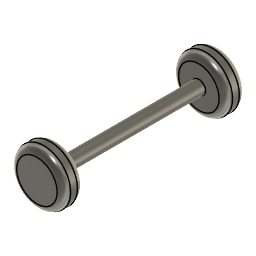
Dozer and Engine Assembly (Autodesk Fusion 360 archive; units mm, degrees)
design "Wheels"
part number: 2026-03-04-16-00-43-502
Autodesk Fusion 360 part; units mm, degrees
note: some values were not read from the file. Set by a fixed rule: which face or edge a step refers to.
sketch "Sketch1" plane through (0, 0, 0) normal (0, 1, 0) x (1, 0, 0)
  circle A0 centre (0, 0) radius 2.54
  dimension "d1" = 5.08
  constraint coincident A0.centre origin
  measures "d1" diameter of A0
extrude "Extrude1" add sketch "Sketch1" along normal mid plane 53.34
sketch "Sketch2" plane through (0, -26.67, 0) normal (0, -1, 0) x (1, 0, 0)
  circle A0 centre (0, 0) radius 2.54
  circle A1 centre (0, 0) radius 10.16
  dimension "d8" = 20.32
  constraint coincident A0.centre A1.centre
  measures "d8" diameter of A1
extrude "Extrude2" add sketch "Sketch2" along normal blind 7.62 contours A0 | A1
sketch "Sketch3" plane through (0, 26.67, 0) normal (0, 1, 0) x (-1, 0, 0)
  circle A0 centre (0, 0) radius 2.54
  circle A1 centre (0, 0) radius 10.16
  dimension "d9" = 20.32
  constraint coincident A0.centre A1.centre
  measures "d9" diameter of A1
extrude "Extrude3" add sketch "Sketch3" along normal blind 7.62 contours A0 | A1
fillet "Fillet1" radius 2.54 3 edges at (-9.4724, -34.29, -3.674) (9.4724, 34.29, -3.674) (-9.4724, -26.67, -3.674) 1 faces at (-10.1474, 29.21, -0.5064)

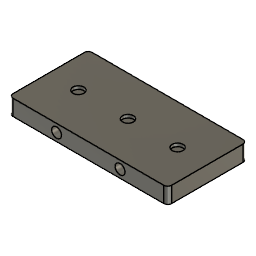
design "Base"
part number: 2026-03-04-09-38-15-257
Autodesk Fusion 360 part; units mm, degrees
sketch "Sketch1" plane through (0, 0, 0) normal (0, 0, 1) x (1, 0, 0)
  line L0 (50.8, -25.4) -> (-50.8, -25.4)
  line L1 (-50.8, -25.4) -> (-50.8, 25.4)
  line L2 (-50.8, 25.4) -> (50.8, 25.4)
  line L3 (50.8, 25.4) -> (50.8, -25.4)
  line L4 (50.8, -25.4) -> (-50.8, 25.4) construction
  line L5 (-50.8, -25.4) -> (50.8, 25.4) construction
  dimension "d2" = 101.6
  dimension "d8" = 50.8
  constraint horizontal L0
  constraint perpendicular L0 L1
  constraint parallel L0 L2
  constraint parallel L1 L3
  constraint coincident L4 origin
  constraint coincident L5 origin
  measures "d2" distance of L1 L3
  measures "d8" distance of L0 L2
extrude "Extrude1" add sketch "Sketch1" against normal blind 10.16
sketch "Sketch2" plane through (0, 0, 0) normal (0, 0, 1) x (-1, 0, 0)
  line L0 (-50.8, -25.4) -> (50.8, -25.4)
  line L1 (50.8, -25.4) -> (50.8, 25.4)
  line L2 (50.8, 25.4) -> (-50.8, 25.4)
  line L3 (-50.8, 25.4) -> (-50.8, -25.4)
  circle A0 centre (31.75, 0) radius 3.5
  circle A1 centre (0, 0) radius 3.5
  circle A2 centre (-31.75, 0) radius 3.5
  line L4 (12.7, -25.4) -> (12.7, 25.4) construction
  dimension "d11" = 7
  dimension "d12" = 19.05
  dimension "d13" = 7
  dimension "d14" = 50.8
  dimension "d15" = 7
  dimension "d16" = 19.05
  dimension "d17" = 25.4
  dimension "d18" = 25.4
  dimension "d19" = 25.4
  dimension "d22" = 38.1
  constraint coincident L0 L4.start
  constraint coincident L2 L4.end
  constraint perpendicular L2 L4
  measures "d11" diameter of A0
  measures "d12" distance of L1 A0.centre
  measures "d13" diameter of A1
  measures "d14" distance of L3 A1.centre
  measures "d15" diameter of A2
  measures "d16" distance of L3 A2.centre
  measures "d17" distance of L2 A0.centre
  measures "d18" distance of L2 A1.centre
  measures "d19" distance of L2 A2.centre
  measures "d22" distance of L1 L4
extrude "Extrude2" cut sketch "Sketch2" against normal blind 2 contours A0 | A1 | A2
sketch "Sketch3" plane through (0, -25.4, 0) normal (0, -1, 0) x (1, 0, 0)
  line L0 (50.8, 0) -> (-50.8, 0)
  line L1 (-50.8, 0) -> (-50.8, -10.16)
  line L2 (-50.8, -10.16) -> (50.8, -10.16)
  line L3 (50.8, -10.16) -> (50.8, 0)
  circle A0 centre (-20.32, -5.08) radius 3.175
  circle A1 centre (20.32, -5.08) radius 3.175
  dimension "d23" = 30.48
  dimension "d24" = 30.48
  dimension "d25" = 6.35
  dimension "d26" = 6.35
  dimension "d27" = 5.08
  dimension "d28" = 5.08
  measures "d23" distance of L1 A0.centre
  measures "d24" distance of L3 A1.centre
  measures "d25" diameter of A0
  measures "d26" diameter of A1
  measures "d27" distance of L0 A0.centre
  measures "d28" distance of L0 A1.centre
extrude "Extrude3" cut sketch "Sketch3" against normal through all contours A0 | A1
fillet "Fillet1" radius 2.54 4 edges at (-50.8, -25.4, -5.08) (-50.8, 25.4, -5.08) (50.8, -25.4, -5.08) (50.8, 25.4, -5.08)

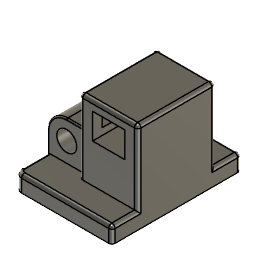
design "Front Dozer Seat"
part number: 2026-03-22-23-02-17-136
Autodesk Fusion 360 part; units mm, degrees
sketch "Sketch1" plane through (0, 0, 0) normal (0, 0, 1) x (1, 0, 0)
  line L0 (19.05, -25.4) -> (-19.05, -25.4)
  line L1 (-19.05, -25.4) -> (-19.05, 25.4)
  line L2 (-19.05, 25.4) -> (19.05, 25.4)
  line L3 (19.05, 25.4) -> (19.05, -25.4)
  line L4 (19.05, -25.4) -> (-19.05, 25.4) construction
  line L5 (-19.05, -25.4) -> (19.05, 25.4) construction
  dimension "d1" = 38.1
  dimension "d2" = 50.8
  constraint horizontal L0
  constraint perpendicular L0 L1
  constraint parallel L0 L2
  constraint parallel L1 L3
  constraint coincident L4 origin
  constraint coincident L5 origin
  measures "d1" distance of L1.end L2.end
  measures "d2" distance of L0.end L1.end
extrude "Extrude1" add sketch "Sketch1" along normal blind 6.35
sketch "Sketch2" plane through (0, 0, 6.35) normal (0, 0, 1) x (-1, 0, 0)
  line L0 (-19.05, -25.4) -> (19.05, -25.4)
  line L1 (19.05, -25.4) -> (19.05, 25.4)
  line L2 (19.05, 25.4) -> (-19.05, 25.4)
  line L3 (-19.05, 25.4) -> (-19.05, -25.4)
  line L4 (19.05, -12.7) -> (3.81, -12.7)
  line L5 (3.81, -12.7) -> (3.81, 12.7)
  line L6 (3.81, 12.7) -> (19.05, 12.7)
  line L7 (19.05, 12.7) -> (19.05, -12.7)
  line L8 (-19.05, -15.24) -> (3.81, -15.24)
  line L9 (3.81, -15.24) -> (3.81, 15.24)
  line L10 (3.81, 15.24) -> (-19.05, 15.24)
  line L11 (-19.05, 15.24) -> (-19.05, -15.24)
  dimension "d5" = 15.24
  dimension "d6" = 25.4
  dimension "d7" = 12.7
  dimension "d9" = 10.16
  dimension "d14" = 10.16
  constraint horizontal L4
  constraint vertical L5
  constraint horizontal L6
  constraint vertical L7
  constraint coincident L1 L4.start
  constraint horizontal L8
  constraint vertical L9
  constraint horizontal L10
  constraint vertical L11
  constraint coincident L3 L8.start
  constraint collinear L5 L9
  measures "d5" distance of L7 L9
  measures "d6" distance of L4 L6
  measures "d7" distance of L0 L4
  measures "d9" distance of L0 L8
  measures "d14" distance of L2 L10
extrude "Extrude2" add sketch "Sketch2" along normal blind 15.24 contours L1 L4 L5 L6 L7 L9
extrude "Extrude3" add sketch "Sketch2" along normal blind 29.21 contours L3 L5 L8 L9 L10 L11
sketch "Sketch3" plane through (0, -12.7, 0) normal (0, -1, 0) x (1, 0, 0)
  line L0 (-19.05, 6.35) -> (-3.81, 6.35)
  line L1 (-3.81, 6.35) -> (-3.81, 21.59)
  line L2 (-3.81, 21.59) -> (-19.05, 21.59)
  line L3 (-19.05, 21.59) -> (-19.05, 6.35)
  circle A0 centre (-11.43, 13.97) radius 3.937
  dimension "d15" = 7.874
  dimension "d16" = 7.62
  dimension "d17" = 7.62
  measures "d15" diameter of A0
  measures "d16" distance of L2 A0.centre
  measures "d17" distance of L3 A0.centre
extrude "Extrude4" cut sketch "Sketch3" against normal through all contours A0
fillet "Fillet1" radius 2.54 2 edges at (-19.05, -25.4, 3.175) (-19.05, 25.4, 3.175)
fillet "Fillet2" radius 1.27 6 edges at (1.27, 25.4, 6.35) (-18.3061, 24.6561, 6.35) (-19.05, 17.78, 6.35) (-19.05, -17.78, 6.35) (-18.3061, -24.6561, 6.35) (1.27, -25.4, 6.35)
fillet "Fillet3" radius 7.62 1 edges at (-19.05, 0, 21.59)
fillet "Fillet4" radius 1.27 14 edges at (-3.81, 15.24, 20.955) (7.62, 15.24, 35.56) (-3.81, 0, 35.56) (7.62, -15.24, 35.56) (-3.81, -15.24, 20.955) (19.05, 0, 35.56) (19.05, -15.24, 20.955) (19.05, 15.24, 20.955) (19.05, -25.4, 2.54) (19.05, -25.028, 5.978) (19.05, -19.685, 6.35) (19.05, 19.685, 6.35) (19.05, 25.028, 5.978) (19.05, 25.4, 2.54)
fillet "Fillet5" radius 0.508 6 edges at (-7.62, 12.7, 21.59) (-16.8182, 12.7, 19.3582) (-19.05, 12.7, 9.525) (-19.05, -12.7, 9.525) (-16.8182, -12.7, 19.3582) (-7.62, -12.7, 21.59)
sketch "Sketch4" plane through (0, 15.24, 0) normal (0, 1, 0) x (-1, 0, 0)
  line L0 (2.54, 6.35) -> (2.54, 34.29)
  line L1 (2.54, 34.29) -> (-17.78, 34.29)
  line L2 (-17.78, 34.29) -> (-17.78, 6.35)
  line L3 (-17.78, 6.35) -> (2.54, 6.35)
  line L4 (-13.97, 31.75) -> (-1.27, 31.75)
  line L5 (-1.27, 31.75) -> (-1.27, 21.59)
  line L6 (-1.27, 21.59) -> (-13.97, 21.59)
  line L7 (-13.97, 21.59) -> (-13.97, 31.75)
  dimension "d29" = 3.81
  dimension "d30" = 3.81
  dimension "d31" = 2.54
  dimension "d32" = 10.16
  constraint horizontal L4
  constraint vertical L5
  constraint horizontal L6
  constraint vertical L7
  measures "d29" distance of L2 L7
  measures "d30" distance of L0 L5
  measures "d31" distance of L1 L4
  measures "d32" distance of L4 L6
extrude "Extrude5" cut sketch "Sketch4" against normal through all contours L4 L5 L6 L7
sketch "Sketch5" plane through (-3.81, 0, 0) normal (-1, 0, 0) x (0, -1, 0)
  line L0 (13.97, 6.35) -> (13.97, 34.29)
  line L1 (13.97, 34.29) -> (-13.97, 34.29)
  line L2 (-13.97, 34.29) -> (-13.97, 6.35)
  line L3 (-13.97, 6.35) -> (-12.7, 6.35)
  line L4 (-12.7, 6.35) -> (-12.7, 21.082)
  arc A0 (-12.192, 21.59) -> (-12.7, 21.082) centre (-12.192, 21.082) ccw
  line L5 (-12.192, 21.59) -> (12.192, 21.59)
  arc A1 (12.7, 21.082) -> (12.192, 21.59) centre (12.192, 21.082) ccw
  line L6 (12.7, 21.082) -> (12.7, 6.35)
  line L7 (12.7, 6.35) -> (13.97, 6.35)
  line L8 (-11.43, 33.02) -> (11.43, 33.02)
  line L9 (11.43, 33.02) -> (11.43, 24.2438)
  line L10 (11.43, 24.2438) -> (-11.43, 24.2438)
  line L11 (-11.43, 24.2438) -> (-11.43, 33.02)
  constraint horizontal L8
  constraint vertical L9
  constraint horizontal L10
  constraint vertical L11
extrude "Extrude6" cut sketch "Sketch5" against normal up to surface (17.78 mm away) contours L8 L9 L10 L11
sketch "Sketch6" plane through (0, 0, 0) normal (0, 0, -1) x (1, 0, 0)
  arc A0 (19.05, 24.13) -> (17.78, 25.4) centre (17.78, 24.13) ccw
  line L0 (17.78, 25.4) -> (-16.51, 25.4)
  arc A1 (-16.51, 25.4) -> (-19.05, 22.86) centre (-16.51, 22.86) ccw
  line L1 (-19.05, 22.86) -> (-19.05, -22.86)
  arc A2 (-19.05, -22.86) -> (-16.51, -25.4) centre (-16.51, -22.86) ccw
  line L2 (-16.51, -25.4) -> (17.78, -25.4)
  arc A3 (17.78, -25.4) -> (19.05, -24.13) centre (17.78, -24.13) ccw
  line L3 (19.05, -24.13) -> (19.05, 24.13)
  circle A4 centre (0, 0) radius 3.5
  dimension "d36" = 7
  constraint coincident A4.centre origin
  measures "d36" diameter of A4
extrude "Extrude7" cut sketch "Sketch6" against normal blind 2 contours A4

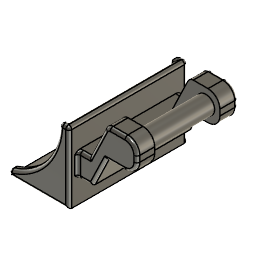
design "Dozer"
part number: 2026-03-22-23-28-42-444
Autodesk Fusion 360 part; units mm, degrees
sketch "Sketch1" plane through (0, 0, 0) normal (0, 1, 0) x (1, 0, 0)
  line L0 (-25.4, 0) -> (0, 0)
  line L1 (0, 0) -> (0, -30.48)
  line L2 (0, -30.48) -> (-2.54, -30.48)
  arc A0 (-2.54, -30.48) -> (-25.4, 0) centre (-33.6513, -30.001) ccw
  dimension "d1" = 30.48
  dimension "d2" = 2.54
  dimension "d5" = 25.4
  dimension "d6" = 31.115
  constraint coincident L0.end L1.start
  constraint horizontal L0
  constraint perpendicular L0 L1
  constraint perpendicular L1 L2
  constraint coincident L0.start A0.end
  measures "d1" distance of L0.end L1.end
  measures "d2" distance of L1.end L2.end
  measures "d5" distance of L0.start L0.end
  measures "d6" radius of A0
extrude "Extrude1" add sketch "Sketch1" along normal mid plane 50.8
sketch "Sketch2" plane through (0, 0, 0) normal (1, 0, 0) x (0, 1, 0)
  line L0 (-25.4, 0) -> (25.4, 0)
  line L1 (25.4, 0) -> (25.4, 30.48)
  line L2 (25.4, 30.48) -> (-25.4, 30.48)
  line L3 (-25.4, 30.48) -> (-25.4, 0)
  line L4 (-13.97, 20.32) -> (13.97, 20.32)
  line L5 (13.97, 20.32) -> (13.97, 10.16)
  line L6 (13.97, 10.16) -> (-13.97, 10.16)
  line L7 (-13.97, 10.16) -> (-13.97, 20.32)
  dimension "d9" = 27.94
  dimension "d10" = 10.16
  dimension "d11" = 10.16
  dimension "d12" = 11.43
  constraint horizontal L4
  constraint vertical L5
  constraint horizontal L6
  constraint vertical L7
  measures "d9" distance of L4.start L4.end
  measures "d10" distance of L4.start L6.end
  measures "d11" distance of L0 L6
  measures "d12" distance of L3 L7
extrude "Extrude2" add sketch "Sketch2" along normal blind 10.16 contours L4 L5 L6 L7
sketch "Sketch3" plane through (0, -13.97, 0) normal (0, -1, 0) x (1, 0, 0)
  line L0 (0, 20.32) -> (0, 10.16)
  line L1 (0, 10.16) -> (10.16, 10.16)
  line L2 (10.16, 10.16) -> (10.16, 20.32)
  line L3 (10.16, 20.32) -> (0, 20.32)
  line L4 (5.08, 20.32) -> (12.4091, 35.56)
  line L5 (12.4091, 35.56) -> (25.4, 35.56)
  line L6 (25.4, 35.56) -> (25.4, 22.86)
  line L7 (25.4, 22.86) -> (12.4576, 22.86)
  line L8 (12.4576, 22.86) -> (6.35, 10.16)
  line L9 (5.08, 20.32) -> (0, 20.32)
  line L10 (0, 10.16) -> (6.35, 10.16)
  line L11 (0, 20.32) -> (0, 10.16)
  line L12 (-25.4, 0) -> (0, 0)
  dimension "d22" = 25.4
  dimension "d23" = 22.86
  dimension "d24" = 12.7
  constraint perpendicular L0 L5
  constraint perpendicular L5 L6
  constraint perpendicular L6 L7
  constraint parallel L4 L8
  constraint midpoint L3 L4.start
  constraint coincident L0.start L3.end
  constraint coincident L0.end L1.start
  constraint perpendicular L0 L10
  measures "d22" distance of L6 L11
  measures "d23" distance of L7 L12
  measures "d24" distance of L5 L7
extrude "Extrude3" add sketch "Sketch3" along normal blind 7.62 contours L0 L1 L2 L3 L8 L9 L10 L11 | L2 L3 L4 L5 L6 L7 L8
mirror "Mirror1" about plane through (0, 0, 0) normal (0, 1, 0) of "Extrude3"
sketch "Sketch4" plane through (0, -13.97, 0) normal (0, 1, 0) x (-1, 0, 0)
  line L0 (-10.16, 20.32) -> (-5.08, 20.32)
  line L1 (-5.08, 20.32) -> (-12.4091, 35.56)
  line L2 (-12.4091, 35.56) -> (-25.4, 35.56)
  line L3 (-25.4, 35.56) -> (-25.4, 22.86)
  line L4 (-25.4, 22.86) -> (-12.4576, 22.86)
  line L5 (-12.4576, 22.86) -> (-10.16, 18.0824)
  line L6 (-10.16, 18.0824) -> (-10.16, 20.32)
  circle A0 centre (-19.346, 29.21) radius 3.81
  line L7 (-32.4673, 29.21) -> (-5.1482, 29.21) construction
  dimension "d19" = 7.62
  constraint perpendicular L3 L7
  constraint coincident A0.centre L7
  measures "d19" diameter of A0
extrude "Extrude4" add sketch "Sketch4" along normal up to surface (27.94 mm away) contours A0
extrude "Extrude5" cut 1 faces at (8.89, -13.97, 12.8008) along direction (0, 1, 0) through all
sketch "Sketch5" plane through (0, -25.4, 0) normal (0, -1, 0) x (1, 0, 0)
  line L0 (0, 30.48) -> (-2.54, 30.48)
  arc A0 (-25.4, 0) -> (-2.54, 30.48) centre (-33.6513, 30.001) ccw
  line L1 (-25.4, 0) -> (0, 0)
  line L2 (0, 0) -> (0, 30.48)
  line L3 (0, 0) -> (-25.4, 0)
  line L4 (-25.4, 0) -> (-25.4, 2.54)
  line L5 (0, 0) -> (0, 30.48)
  line L6 (0, 30.48) -> (-3.81, 30.48)
  arc A1 (-25.4, 2.54) -> (-3.81, 30.48) centre (-33.6723, 31.2438) ccw
  constraint coincident L1.end L2.start
  constraint coincident A0.start L1.start
  constraint perpendicular L3 L4
  constraint coincident L0.start L2.end
  constraint perpendicular L2 L6
  constraint tangent A0 A1
extrude "Extrude6" add sketch "Sketch5" against normal blind 2.54
mirror "Mirror2" about plane through (0, 0, 0) normal (0, 1, 0) of "Extrude6"
fillet "Fillet1" radius 1.27 2 edges at (-25.4, -24.13, 2.54) (-25.4, 24.13, 2.54) 3 faces at (-0.8467, -7.62, 30.48) (-1.7311, -25.4, 17.5693) (-1.7311, 25.4, 17.5693)
fillet "Fillet2" radius 1.27 2 faces at (16.7556, 21.59, 31.3267) (16.7556, -21.59, 31.3267)
fillet "Fillet3" radius 5.08 8 edges at (25.4, -17.145, 35.56) (25.028, -21.218, 35.188) (25.4, -17.145, 22.86) (25.028, -21.218, 23.232) (25.4, 17.145, 22.86) (25.028, 21.218, 23.232) (25.4, 17.145, 35.56) (25.028, 21.218, 35.188)
fillet "Fillet4" radius 2.54 4 edges at (12.4091, 17.145, 35.56) (12.643, 21.218, 35.188) (12.4091, -17.145, 35.56) (12.643, -21.218, 35.188)
